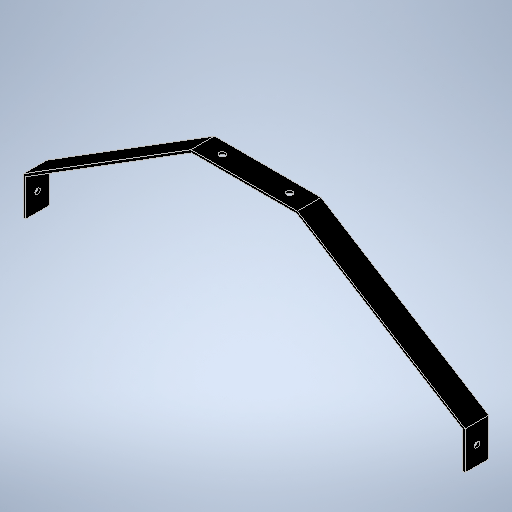
# Autodesk Inventor part: A-MainGear
Saved by Autodesk Inventor 2025.3 (Build 293356000, 356)
## iProperties
Created: 2025-07-09
Part Number: A-MainGear
Material: Generic
Document SubType Name: Modeling
Designer: steve
Density: 1 g/cm^3
Appearance: Anodized - Black
Author: steve
Autodesk Inventor part; units mm, degrees
ref_plane "YZ Plane" through (0, 0, 0) normal (1, 0, 0) x (0, 1, 0)
ref_plane "XZ Plane" through (0, 0, 0) normal (0, 1, 0) x (-1, 0, 0)
ref_plane "XY Plane" through (0, 0, 0) normal (0, 0, 1) x (1, 0, 0)
sketch "Sketch1" plane through (0, 0, 0) normal (0, 0, 1) x (1, 0, 0)
  line L0 (0, 0) -> (-1.35, 0)
  line L1 (0, 0) -> (0, 20)
  line L2 (0, 20) -> (90.49, 20) construction
  line L3 (90.49, 20) -> (90.49, 76.5) construction
  line L4 (90.49, 76.5) -> (0, 20)
  line L5 (90.49, 76.5) -> (147.79, 76.5)
  line L6 (119.14, 76.5) -> (119.14, 94.3884) construction
  line L7 (-1.35, 0) -> (-1.35, 20.7486)
  line L8 (-1.35, 20.7486) -> (90.1032, 77.85)
  line L9 (119.14, 77.85) -> (90.1032, 77.85)
  line L10 (238.28, 0) -> (239.63, 0)
  line L11 (238.28, 0) -> (238.28, 20)
  line L12 (147.79, 76.5) -> (238.28, 20)
  line L13 (147.79, 76.5) -> (90.49, 76.5)
  line L14 (239.63, 0) -> (239.63, 20.7486)
  line L15 (239.63, 20.7486) -> (148.1768, 77.85)
  line L16 (119.14, 77.85) -> (148.1768, 77.85)
  dimension "d0" = 1.35
  dimension "d1" = 20
  dimension "d2" = 90.49
  dimension "d3" = 56.5
  dimension "d4" = 57.3
  dimension "d5" = 1.35
  dimension "d6" = 1.35
  constraints: 34 end point, 7 symmetric about line, 3 horizontal, 3 vertical, 2 perpendicular, 1 midpoint, 1 parallel, 1 point on line
  measures "d0" distance of L0.start L0.end
  measures "d1" distance of L0.start L1.end
  measures "d2" distance of L1.end L2.end
  measures "d3" distance of L2.end L3.end
  measures "d4" distance of L3.end L5.end
  measures "d5" distance between parallel lines of L8 L4
  measures "d6" distance between parallel lines of L9 L5
extrude "Extrusion1" add sketch "Sketch1" along normal mid plane 12.9
sketch "Sketch2" plane through (90.1032, 77.85, 6.45) normal (0, 1, 0) x (1, 0, 0)
  circle A0 centre (10.7168, 6.45) radius 1.75
  line L0 (10.7168, 6.45) -> (47.3568, 6.45)
  circle A1 centre (47.3568, 6.45) radius 1.75
  line L1 (0, 12.9) -> (58.0737, 12.9) projected
  point P0 (-90.1032, 6.45)
  point P1 (29.0368, 12.9)
  point P2 (29.0368, 6.45)
  dimension "d9" = 3.5
  dimension "d10" = 36.64
  dimension "d11" = 3.5
  dimension "d12" = 0
  constraints: 2 centre point, 2 end point, 2 midpoint, 1 coincident, 1 horizontal
  measures "d9" diameter of A0
  measures "d10" distance of L0.start L0.end
  measures "d11" diameter of A1
  measures "d12" horizontal distance of point (29.037, 12.9) point (29.037, 6.45)
extrude "Extrusion2" cut sketch "Sketch2" against normal blind 12.9
sketch "Sketch4" plane through (239.63, 0, 6.45) normal (1, 0, 0) x (0, 0, -1)
  circle A0 centre (6.45, 10) radius 1.5
  point P0 (6.45, 0)
  dimension "d15" = 3
  constraints: 1 centre point
  measures "d15" diameter of A0
extrude "Extrusion3" cut sketch "Sketch4" against normal through all
body "Solid1"
